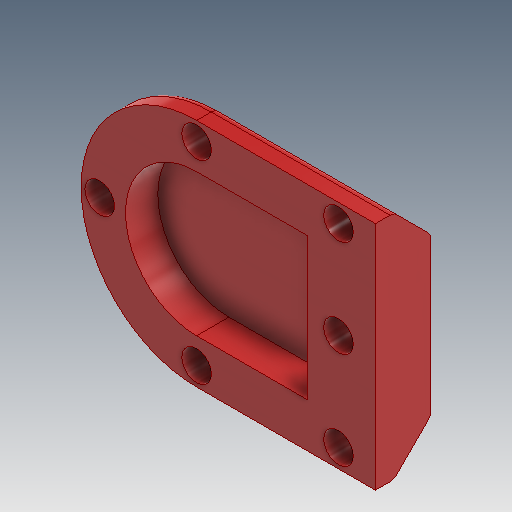
# Autodesk Inventor part: Cover part of robot arm
Saved by Autodesk Inventor 2020.3 (Build 243373010, 373A)
## iProperties
Created: 2021-04-23
Part Number: Cover part of robot arm
Material: Steel, Alloy
Document SubType Name: Modeling
Designer: marti
Density: 7.73 g/cm^3
Appearance: Red
Mass: 2513.31 g
Surface Area: 557.813 cm^2
Volume: 325.137 cm^3
Author: marti
Autodesk Inventor part; units mm, degrees
ref_plane "YZ Plane" through (0, 0, 0) normal (1, 0, 0) x (0, 1, 0)
ref_plane "XZ Plane" through (0, 0, 0) normal (0, 1, 0) x (-1, 0, 0)
ref_plane "XY Plane" through (0, 0, 0) normal (0, 0, 1) x (1, 0, 0)
sketch "Sketch6" plane through (0, 0, 0) normal (0, 0, 1) x (1, 0, 0)
  line L0 (60, 38.5) -> (60, -38.5)
  line L1 (60, -38.5) -> (0, -38.5)
  arc A0 (0, 38.5) -> (0, -38.5) centre (0, 0) ccw
  line L2 (0, 38.5) -> (60, 38.5)
  circle A1 centre (0, -52.5) radius 8.025
  circle A2 centre (-52.5, 0) radius 8.025
  circle A3 centre (0, 52.5) radius 8.025
  circle A4 centre (76.8233, 52.5) radius 8.025
  circle A5 centre (76.8233, 0) radius 8.025
  line L3 (0, 62.5) -> (96.8233, 62.5)
  arc A6 (0, 62.5) -> (0, -62.5) centre (0, 0) ccw
  line L4 (96.8233, -62.5) -> (0, -62.5)
  line L5 (96.8233, 62.5) -> (96.8233, -62.5)
  circle A7 centre (76.8233, -52.5) radius 8.025
  point P0 (0, 0)
  point P1 (102.5, 0)
  dimension "d42" = 16.05
  dimension "d43" = 60
  dimension "d44" = 38.5
  constraints: 12 end point, 8 centre point, 5 equal radius, 4 point on circle, 2 horizontal, 1 coincident, 1 vertical, 1 other
  measures "d42" diameter of A7
  measures "d43" distance from line of point (0, 0) L0
  measures "d44" distance from line of point (0, 0) L1
extrude "Extrusion8" add sketch "Sketch6" against normal mid plane 30
chamfer "Chamfer3" distance 20 angle 45 3 edges at (-62.5, 0, -15) (48.4116, 62.5, -15) (48.4116, -62.5, -15)
fillet "Fillet3" radius 5 3 edges at (48.4116, 42.5, -15) (48.4116, -42.5, -15) (-42.5, 0, -15)
sketch "Sketch7" plane through (0, 0, -15) normal (0, 0, -1) x (-1, 0, 0)
  line L0 (0, -40.4289) -> (-96.8233, -40.4289) projected
  arc A0 (0, -40.4289) -> (0, 40.4289) centre (0, 0) ccw projected
  line L1 (-96.8233, 40.4289) -> (0, 40.4289) projected
  line L2 (-96.8233, 40.4289) -> (-96.8233, -40.4289) projected
  circle A1 centre (-76.8233, 0) radius 8.025 projected
  line L3 (-60, 38.5) -> (0, 38.5) projected
  arc A2 (0, -38.5) -> (0, 38.5) centre (0, 0) ccw projected
  line L4 (0, -38.5) -> (-60, -38.5) projected
  line L5 (-60, -38.5) -> (-60, 38.5) projected
  point P0 (0, 0)
extrude "Extrusion10" add sketch "Sketch7" against normal blind 12.5 contours L3 A2 L4 L5
fillet "Fillet4" radius 5 3 edges at (-62.5, 0, 5) (48.4116, -62.5, 5) (48.4116, 62.5, 5)
body "Solid3"
